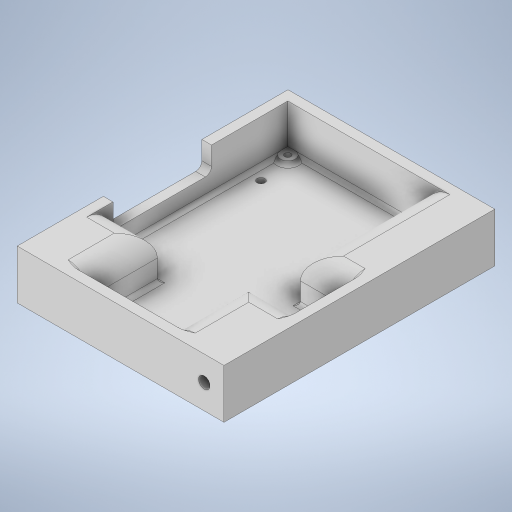
# Autodesk Inventor part: top
Saved by Autodesk Inventor 2024 (Build 280153000, 153)
## iProperties
Created: 2023-11-27
Part Number: top
Material: Generic
Document SubType Name: Modeling
Designer: CJ110
Density: 1 g/cm^3
Appearance: Default
Author: CJ110
Autodesk Inventor part; units mm, degrees
ref_plane "YZ Plane" through (0, 0, 0) normal (1, 0, 0) x (0, 1, 0)
ref_plane "XZ Plane" through (0, 0, 0) normal (0, 1, 0) x (-1, 0, 0)
ref_plane "XY Plane" through (0, 0, 0) normal (0, 0, 1) x (1, 0, 0)
sketch "Sketch1" plane through (0, 0, 0) normal (0, 1, 0) x (-1, 0, 0)
  line L0 (-42.5196, -32.4485) -> (42.5196, -32.4485) construction
  line L1 (42.5196, -32.4485) -> (42.5196, 32.4485) construction
  line L2 (42.5196, 32.4485) -> (-42.5196, 32.4485) construction
  line L3 (-42.5196, 32.4485) -> (-42.5196, -32.4485) construction
  line L4 (-42.5196, -32.4485) -> (42.5196, 32.4485) construction
  line L5 (42.5196, -32.4485) -> (-42.5196, 32.4485) construction
  circle A0 centre (42.5196, 32.4485) radius 3.81
  circle A1 centre (42.5196, 32.4485) radius 1.5875
  circle A2 centre (-42.5196, 32.4485) radius 3.81
  circle A3 centre (-42.5196, 32.4485) radius 1.5875
  circle A4 centre (-42.5196, -32.4485) radius 3.81
  circle A5 centre (-42.5196, -32.4485) radius 1.5875
  circle A6 centre (42.5196, -32.4485) radius 3.81
  circle A7 centre (42.5196, -32.4485) radius 3.81
  circle A8 centre (42.5196, -32.4485) radius 1.5875
  line L6 (45.085, -35.052) -> (-45.085, -35.052) construction
  line L7 (-45.085, -35.052) -> (-45.085, 35.052) construction
  line L8 (-45.085, 35.052) -> (45.085, 35.052) construction
  line L9 (45.085, 35.052) -> (45.085, -35.052) construction
  line L10 (45.085, -35.052) -> (-45.085, 35.052) construction
  line L11 (-45.085, -35.052) -> (45.085, 35.052) construction
  line L12 (-83.185, 60.452) -> (46.3296, 60.452)
  line L13 (46.3296, 60.452) -> (46.3296, -36.2585)
  line L14 (46.3296, -36.2585) -> (-83.185, -36.2585)
  line L15 (-83.185, -36.2585) -> (-83.185, 60.452)
  line L16 (-88.2777, 65.4368) -> (51.4223, 65.4368)
  line L17 (51.4223, 65.4368) -> (51.4223, -41.2433)
  line L18 (51.4223, -41.2433) -> (-88.2777, -41.2433)
  line L19 (-88.2777, -41.2433) -> (-88.2777, 65.4368)
  line L20 (-19.685, 60.452) -> (-19.685, 36.2585)
  line L21 (-46.3296, -10.8585) -> (-83.185, -10.8585)
  line L22 (-42.5196, 36.2585) -> (-42.5196, 60.452)
  line L23 (-46.3296, -10.8585) -> (-46.3296, -36.2585)
  line L24 (-19.685, 36.2585) -> (46.3296, 36.2585)
  line L25 (-42.5196, 32.4485) -> (-46.3296, 32.4485) construction
  line L26 (-42.5196, 32.4485) -> (-42.5196, 36.2585) construction
  line L27 (-46.3296, 32.4485) -> (-83.185, 32.4485)
  line L28 (46.3296, 60.452) -> (51.4223, 60.452) construction
  line L29 (46.3296, 60.452) -> (46.3296, 65.4368) construction
  line L30 (-83.185, -36.2585) -> (-83.185, -41.2433) construction
  line L31 (-83.185, -36.2585) -> (-88.2777, -36.2585) construction
  point P0 (0, 0)
  point P1 (-39.7379, 35.052)
  point P2 (-45.085, 29.6316)
  point P3 (46.3296, 32.4485)
  point P4 (39.7379, 35.052)
  point P5 (-45.085, -29.6316)
  point P6 (-42.5196, -36.2585)
  point P7 (-83.185, 36.2585)
  point P8 (-45.085, 35.2654)
  point P9 (-39.7379, -35.052)
  point P10 (39.7379, -35.052)
  point P11 (45.085, -29.6316)
  point P12 (45.085, 29.6316)
  point P13 (42.5196, -36.2585)
  point P14 (46.3296, -32.4485)
  point P15 (39.7379, 35.052)
  point P16 (-45.085, -29.6316)
  point P17 (-46.3296, -32.4485)
  point P18 (42.5196, 36.2585)
  dimension "d5" = 7.62
  dimension "d7" = 7.62
  dimension "d4" = 7.62
  dimension "d6" = 7.62
  dimension "d8" = 3.175
  dimension "d9" = 3.175
  dimension "d10" = 3.175
  dimension "d11" = 3.175
  dimension "d18" = 70.104
  dimension "d19" = 90.17
  dimension "d23" = 85.0392
  dimension "d24" = 64.897
  dimension "d25" = 38.1
  dimension "d26" = 25.4
  dimension "d31" = 25.4
  dimension "d32" = 25.4
  dimension "d41" = 139.7
  dimension "d43" = 106.68
  constraints: 64 end point, 14 point on line, 13 perpendicular, 10 parallel, 9 coincident, 7 centre point, 6 horizontal, 4 midpoint, 2 point on circle, 2 tangent, 1 collinear, 1 concentric, 1 vertical, 6 other
  measures "d4" diameter of A2
  measures "d6" diameter of A6
  measures "d8" diameter of A3
  measures "d9" diameter of A1
  measures "d10" diameter of A8
  measures "d11" diameter of A5
  measures "d18" distance of L6.end L7.end
  measures "d19" distance of L6.start L6.end
  measures "d23" distance of L1.end L2.end
  measures "d24" distance of L2.end L0.start
  measures "d25" distance between parallel lines of L7 L15
  measures "d26" distance between parallel lines of L8 L12
  measures "d31" distance between parallel lines of L7 L20
  measures "d32" distance between parallel lines of L14 L21
  measures "d41" distance between parallel lines of L17 L19
  measures "d43" distance between parallel lines of L16 L18
extrude "Extrusion5" add sketch "Sketch1" against normal blind 3.175 contours L13 A6 L14 A4 L23 L21 L15 L27 A2 L22 L12 L20 L24 A0 | A0 L24 L13 | L24 L20 L12 L13 | L13 L14 A6 | L14 L23 A4 | L22 A2 L27 L15 L12 | L23 L14 L15 L21 | L16 L17 L18 L19
extrude "Extrusion2" add sketch "Sketch1" against normal blind 5.08 contours A0 | A0 L24 L13 | A6 | L13 L14 A6 | L14 L23 A4 | A4 | A2
extrude "Extrusion4" add sketch "Sketch1" against normal blind 25.4 contours L24 L20 L12 L13 | L22 A2 L27 L15 L12 | L23 L14 L15 L21 | L16 L17 L18 L19
fillet "Fillet1" radius 11.1125 1 edges at (83.185, -3.175, 10.795)
fillet "Fillet2" radius 11.1125 1 edges at (31.1023, -3.175, 60.452)
fillet "Fillet3" radius 11.1125 6 edges at (42.5196, -25.4, 48.3553) (64.7573, -25.4, -10.8585) (46.3296, -25.4, -23.5585) (-13.3223, -25.4, 36.2585) (19.685, -25.4, 48.3552) (64.7573, -25.4, 32.4485)
fillet "Fillet4" radius 1.905 19 edges at (-46.3296, -3.175, 0) (-39.8255, -3.175, -29.7544) (39.8255, -3.175, -29.7544) (46.3296, -3.175, -21.6535) (79.9302, -6.4298, -10.8585) (83.185, -22.1452, -14.1133) (59.2011, -3.175, -10.8585) (-11.4173, -3.175, 36.2585) (19.685, -6.4298, 57.1972) (16.4302, -22.1452, 60.452) (19.685, -3.175, 42.799) (39.8255, -3.175, 29.7544) (42.5196, -6.4298, 57.1972) (45.7744, -22.1452, 60.452) (42.5196, -3.175, 42.799) (79.9302, -6.4298, 32.4485) (59.2011, -3.175, 32.4485) (0, -3.175, -36.2585) (-39.8255, -3.175, 29.7544)
sketch "Sketch4" plane through (0, 0, 0) normal (0, 1, 0) x (1, 0, 0)
  line L0 (88.2777, -65.4368) -> (-51.4223, -65.4368) construction
  line L1 (-51.4223, -65.4368) -> (-51.4223, 41.2433) construction
  line L2 (-51.4223, 41.2433) -> (88.2777, 41.2433) construction
  line L3 (88.2777, 41.2433) -> (88.2777, -65.4368) construction
  line L4 (50.5528, -6.0666) -> (50.5528, -17.9953)
  line L5 (50.5528, -17.9953) -> (48.6146, -18.1269)
  spline S0 degree 2 poles (48.6146, -18.1269) (47.1668, -18.1269) (46.3173, -17.2296) knots 0 0 0 1 1 1
  spline S1 degree 2 poles (46.3173, -17.2296) (45.4798, -16.3203) (45.4798, -14.9324) knots 0 0 0 1 1 1
  spline S2 degree 2 poles (45.4798, -14.9324) (45.4798, -13.1855) (46.9993, -12.4198) knots 0 0 0 1 1 1
  spline S3 degree 2 poles (46.9993, -12.4198) (44.5585, -11.8694) (44.5585, -9.2492) knots 0 0 0 1 1 1
  spline S4 degree 2 poles (44.5585, -9.2492) (44.5585, -7.9211) (45.3602, -6.928) knots 0 0 0 1 1 1
  spline S5 degree 2 poles (45.3602, -6.928) (46.1738, -5.9349) (47.9924, -5.9349) knots 0 0 0 1 1 1
  spline S6 degree 2 poles (47.9924, -5.9349) (48.6505, -5.9349) (49.4401, -6.0067) knots 0 0 0 1 1 1
  spline S7 degree 2 poles (49.4401, -6.0067) (50.1341, -6.0666) (50.5528, -6.0666) knots 0 0 0 1 1 1
  line L6 (48.483, -11.8216) -> (49.6196, -11.8216)
  line L7 (49.6196, -11.8216) -> (49.6196, -9.7876)
  spline S8 degree 2 poles (49.6196, -9.7876) (49.6196, -7.6579) (49.153, -7.0836) knots 0 0 0 1 1 1
  spline S9 degree 2 poles (49.153, -7.0836) (48.7581, -6.7844) (47.9685, -6.7844) knots 0 0 0 1 1 1
  spline S10 degree 2 poles (47.9685, -6.7844) (46.6404, -6.7844) (46.0661, -7.5502) knots 0 0 0 1 1 1
  spline S11 degree 2 poles (46.0661, -7.5502) (45.5277, -8.3159) (45.5277, -9.3449) knots 0 0 0 1 1 1
  spline S12 degree 2 poles (45.5277, -9.3449) (45.5277, -10.1704) (45.8747, -10.7567) knots 0 0 0 1 1 1
  spline S13 degree 2 poles (45.8747, -10.7567) (46.2456, -11.3549) (46.784, -11.5942) knots 0 0 0 1 1 1
  spline S14 degree 2 poles (46.784, -11.5942) (47.3583, -11.8216) (48.483, -11.8216) knots 0 0 0 1 1 1
  line L8 (51.3784, -17.9953) -> (51.3784, -6.0666)
  spline S15 degree 2 poles (51.3784, -6.0666) (52.3715, -6.0307) (53.7594, -5.9349) knots 0 0 0 1 1 1
  line L9 (53.7594, -5.9349) -> (53.7594, -6.1383)
  spline S16 degree 2 poles (53.7594, -6.1383) (52.3116, -6.5332) (52.3116, -9.2013) knots 0 0 0 1 1 1
  line L10 (52.3116, -9.2013) -> (52.3116, -15.0999)
  spline S17 degree 2 poles (52.3116, -15.0999) (52.3116, -17.445) (53.7594, -17.9235) knots 0 0 0 1 1 1
  line L11 (53.7594, -17.9235) -> (53.7594, -18.1269)
  spline S18 degree 2 poles (53.7594, -18.1269) (52.5868, -18.0193) (51.3784, -17.9953) knots 0 0 0 1 1 1
  line L12 (49.6196, -14.8965) -> (49.6196, -12.6232)
  line L13 (49.6196, -12.6232) -> (48.7462, -12.6232)
  spline S19 degree 2 poles (48.7462, -12.6232) (47.6574, -12.6232) (47.0711, -13.2095) knots 0 0 0 1 1 1
  spline S20 degree 2 poles (47.0711, -13.2095) (46.4729, -13.7957) (46.4729, -14.9084) knots 0 0 0 1 1 1
  spline S21 degree 2 poles (46.4729, -14.9084) (46.4729, -16.0571) (47.119, -16.6553) knots 0 0 0 1 1 1
  spline S22 degree 2 poles (47.119, -16.6553) (47.7531, -17.2416) (48.6385, -17.2416) knots 0 0 0 1 1 1
  spline S23 degree 2 poles (48.6385, -17.2416) (49.1171, -17.2416) (49.4162, -17.0023) knots 0 0 0 1 1 1
  spline S24 degree 2 poles (49.4162, -17.0023) (49.6196, -16.3921) (49.6196, -14.8965) knots 0 0 0 1 1 1
  spline S25 degree 2 poles (44.7619, -6.3896) (43.721, -7.4784) (43.721, -9.1893) knots 0 0 0 1 1 1
  spline S26 degree 2 poles (43.721, -9.1893) (43.721, -11.0199) (44.8098, -12.1446) knots 0 0 0 1 1 1
  spline S27 degree 2 poles (44.8098, -12.1446) (42.6562, -11.3669) (42.6562, -9.2851) knots 0 0 0 1 1 1
  spline S28 degree 2 poles (42.6562, -9.2851) (42.6562, -8.2561) (43.2544, -7.4545) knots 0 0 0 1 1 1
  spline S29 degree 2 poles (43.2544, -7.4545) (43.8526, -6.6528) (44.7619, -6.3896) knots 0 0 0 1 1 1
  spline S30 degree 2 poles (45.3243, -12.7787) (44.6303, -13.6881) (44.6303, -14.9324) knots 0 0 0 1 1 1
  spline S31 degree 2 poles (44.6303, -14.9324) (44.6303, -15.9135) (45.0132, -16.7031) knots 0 0 0 1 1 1
  spline S32 degree 2 poles (45.0132, -16.7031) (45.42, -17.5048) (45.9345, -17.78) knots 0 0 0 1 1 1
  spline S33 degree 2 poles (45.9345, -17.78) (44.8098, -17.5407) (44.2116, -16.8108) knots 0 0 0 1 1 1
  spline S34 degree 2 poles (44.2116, -16.8108) (43.6133, -16.081) (43.6133, -15.1836) knots 0 0 0 1 1 1
  spline S35 degree 2 poles (43.6133, -15.1836) (43.6133, -14.394) (44.1158, -13.6881) knots 0 0 0 1 1 1
  spline S36 degree 2 poles (44.1158, -13.6881) (44.6064, -13.0061) (45.3243, -12.7787) knots 0 0 0 1 1 1
  spline S37 degree 2 poles (29.5189, -12.0968) (29.5189, -10.0029) (30.1531, -8.5672) knots 0 0 0 1 1 1
  spline S38 degree 2 poles (30.1531, -8.5672) (30.7752, -7.1434) (31.9119, -6.4614) knots 0 0 0 1 1 1
  spline S39 degree 2 poles (31.9119, -6.4614) (33.0126, -5.7674) (34.4963, -5.7674) knots 0 0 0 1 1 1
  spline S40 degree 2 poles (34.4963, -5.7674) (36.8533, -5.7674) (38.1455, -7.4545) knots 0 0 0 1 1 1
  spline S41 degree 2 poles (38.1455, -7.4545) (39.4377, -9.1415) (39.4377, -12.0968) knots 0 0 0 1 1 1
  spline S42 degree 2 poles (39.4377, -12.0968) (39.4377, -15.1717) (38.1215, -16.8108) knots 0 0 0 1 1 1
  spline S43 degree 2 poles (38.1215, -16.8108) (36.8054, -18.4261) (34.5202, -18.4261) knots 0 0 0 1 1 1
  spline S44 degree 2 poles (34.5202, -18.4261) (32.211, -18.4261) (30.859, -16.8108) knots 0 0 0 1 1 1
  spline S45 degree 2 poles (30.859, -16.8108) (29.5189, -15.2076) (29.5189, -12.0968) knots 0 0 0 1 1 1
  spline S46 degree 2 poles (30.5838, -12.0848) (30.5838, -17.5048) (34.5202, -17.5048) knots 0 0 0 1 1 1
  spline S47 degree 2 poles (34.5202, -17.5048) (38.3848, -17.5048) (38.3848, -11.9412) knots 0 0 0 1 1 1
  spline S48 degree 2 poles (38.3848, -11.9412) (38.3848, -6.7126) (34.4843, -6.7126) knots 0 0 0 1 1 1
  spline S49 degree 2 poles (34.4843, -6.7126) (30.5838, -6.7126) (30.5838, -12.0848) knots 0 0 0 1 1 1
  spline S50 degree 2 poles (39.0548, -16.9424) (40.2991, -15.0161) (40.2991, -12.013) knots 0 0 0 1 1 1
  spline S51 degree 2 poles (40.2991, -12.013) (40.2991, -9.297) (39.1146, -7.2989) knots 0 0 0 1 1 1
  spline S52 degree 2 poles (39.1146, -7.2989) (41.3999, -8.8065) (41.3999, -12.1207) knots 0 0 0 1 1 1
  spline S53 degree 2 poles (41.3999, -12.1207) (41.3999, -15.5306) (39.0548, -16.9424) knots 0 0 0 1 1 1
  spline S54 degree 2 poles (29.9257, -7.2391) (28.6934, -8.9141) (28.6934, -12.2882) knots 0 0 0 1 1 1
  spline S55 degree 2 poles (28.6934, -12.2882) (28.6934, -15.2674) (29.9138, -16.9305) knots 0 0 0 1 1 1
  spline S56 degree 2 poles (29.9138, -16.9305) (27.5926, -15.5306) (27.5926, -12.1566) knots 0 0 0 1 1 1
  spline S57 degree 2 poles (27.5926, -12.1566) (27.5926, -8.8304) (29.9257, -7.2391) knots 0 0 0 1 1 1
  line L14 (19.1336, -6.0666) -> (19.4208, -6.0666)
  line L15 (19.4208, -6.0666) -> (19.4208, -17.9953)
  line L16 (19.4208, -17.9953) -> (15.3528, -17.9953)
  spline S58 degree 2 poles (15.3528, -17.9953) (14.2281, -17.9953) (13.1513, -18.1269) knots 0 0 0 1 1 1
  spline S59 degree 2 poles (13.1513, -18.1269) (13.1513, -17.9116) (13.1752, -17.3492) knots 0 0 0 1 1 1
  spline S60 degree 2 poles (13.1752, -17.3492) (13.2111, -16.8348) (13.2111, -16.0451) knots 0 0 0 1 1 1
  spline S61 degree 2 poles (13.2111, -16.0451) (13.2111, -15.5545) (13.2709, -15.0401) knots 0 0 0 1 1 1
  line L17 (13.2709, -15.0401) -> (13.5461, -15.0401)
  spline S62 degree 2 poles (13.5461, -15.0401) (13.57, -15.9733) (14.0008, -16.5835) knots 0 0 0 1 1 1
  spline S63 degree 2 poles (14.0008, -16.5835) (14.4554, -17.2057) (15.9151, -17.2057) knots 0 0 0 1 1 1
  line L18 (15.9151, -17.2057) -> (18.4875, -17.2057)
  line L19 (18.4875, -17.2057) -> (18.4875, -9.1056)
  spline S64 degree 2 poles (18.4875, -9.1056) (18.4875, -7.7057) (18.0927, -7.0118) knots 0 0 0 1 1 1
  spline S65 degree 2 poles (18.0927, -7.0118) (17.6979, -6.3058) (16.8723, -6.1383) knots 0 0 0 1 1 1
  line L20 (16.8723, -6.1383) -> (16.8723, -5.9349)
  spline S66 degree 2 poles (16.8723, -5.9349) (18.8704, -6.0666) (19.1336, -6.0666) knots 0 0 0 1 1 1
  line L21 (23.9913, -17.9953) -> (20.2583, -17.9953)
  line L22 (20.2583, -17.9953) -> (20.2583, -6.0666)
  line L23 (20.2583, -6.0666) -> (20.6053, -6.0666)
  spline S67 degree 2 poles (20.6053, -6.0666) (21.3351, -6.0666) (22.7948, -5.9349) knots 0 0 0 1 1 1
  line L24 (22.7948, -5.9349) -> (22.7948, -6.1383)
  spline S68 degree 2 poles (22.7948, -6.1383) (21.8616, -6.3776) (21.5026, -7.0955) knots 0 0 0 1 1 1
  spline S69 degree 2 poles (21.5026, -7.0955) (21.1676, -7.8134) (21.1676, -9.4765) knots 0 0 0 1 1 1
  line L25 (21.1676, -9.4765) -> (21.1676, -17.2057)
  line L26 (21.1676, -17.2057) -> (24.0511, -17.2057)
  spline S70 degree 2 poles (24.0511, -17.2057) (25.1518, -17.2057) (25.6065, -16.751) knots 0 0 0 1 1 1
  spline S71 degree 2 poles (25.6065, -16.751) (26.0612, -16.2964) (26.3603, -15.0401) knots 0 0 0 1 1 1
  line L27 (26.3603, -15.0401) -> (26.6235, -15.0401)
  spline S72 degree 2 poles (26.6235, -15.0401) (26.6355, -15.1956) (26.6355, -15.3631) knots 0 0 0 1 1 1
  spline S73 degree 2 poles (26.6355, -15.3631) (26.6355, -15.5904) (26.5876, -15.9374) knots 0 0 0 1 1 1
  spline S74 degree 2 poles (26.5876, -15.9374) (26.456, -17.1458) (26.456, -18.1269) knots 0 0 0 1 1 1
  spline S75 degree 2 poles (26.456, -18.1269) (25.8578, -18.0552) (24.9604, -18.0312) knots 0 0 0 1 1 1
  line L28 (24.9604, -18.0312) -> (23.9913, -17.9953)
  line L29 (4.8837, -6.0666) -> (5.1708, -6.0666)
  line L30 (5.1708, -6.0666) -> (5.1708, -17.9953)
  line L31 (5.1708, -17.9953) -> (1.1029, -17.9953)
  spline S76 degree 2 poles (1.1029, -17.9953) (-0.0218, -17.9953) (-1.0986, -18.1269) knots 0 0 0 1 1 1
  spline S77 degree 2 poles (-1.0986, -18.1269) (-1.0986, -17.9116) (-1.0747, -17.3492) knots 0 0 0 1 1 1
  spline S78 degree 2 poles (-1.0747, -17.3492) (-1.0388, -16.8348) (-1.0388, -16.0451) knots 0 0 0 1 1 1
  spline S79 degree 2 poles (-1.0388, -16.0451) (-1.0388, -15.5545) (-0.979, -15.0401) knots 0 0 0 1 1 1
  line L32 (-0.979, -15.0401) -> (-0.7038, -15.0401)
  spline S80 degree 2 poles (-0.7038, -15.0401) (-0.6799, -15.9733) (-0.2492, -16.5835) knots 0 0 0 1 1 1
  spline S81 degree 2 poles (-0.2492, -16.5835) (0.2055, -17.2057) (1.6652, -17.2057) knots 0 0 0 1 1 1
  line L33 (1.6652, -17.2057) -> (4.2376, -17.2057)
  line L34 (4.2376, -17.2057) -> (4.2376, -9.1056)
  spline S82 degree 2 poles (4.2376, -9.1056) (4.2376, -7.7057) (3.8428, -7.0118) knots 0 0 0 1 1 1
  spline S83 degree 2 poles (3.8428, -7.0118) (3.4479, -6.3058) (2.6224, -6.1383) knots 0 0 0 1 1 1
  line L35 (2.6224, -6.1383) -> (2.6224, -5.9349)
  spline S84 degree 2 poles (2.6224, -5.9349) (4.6205, -6.0666) (4.8837, -6.0666) knots 0 0 0 1 1 1
  line L36 (9.7413, -17.9953) -> (6.0084, -17.9953)
  line L37 (6.0084, -17.9953) -> (6.0084, -6.0666)
  line L38 (6.0084, -6.0666) -> (6.3553, -6.0666)
  spline S85 degree 2 poles (6.3553, -6.0666) (7.0852, -6.0666) (8.5449, -5.9349) knots 0 0 0 1 1 1
  line L39 (8.5449, -5.9349) -> (8.5449, -6.1383)
  spline S86 degree 2 poles (8.5449, -6.1383) (7.6116, -6.3776) (7.2527, -7.0955) knots 0 0 0 1 1 1
  spline S87 degree 2 poles (7.2527, -7.0955) (6.9177, -7.8134) (6.9177, -9.4765) knots 0 0 0 1 1 1
  line L40 (6.9177, -9.4765) -> (6.9177, -17.2057)
  line L41 (6.9177, -17.2057) -> (9.8012, -17.2057)
  spline S88 degree 2 poles (9.8012, -17.2057) (10.9019, -17.2057) (11.3566, -16.751) knots 0 0 0 1 1 1
  spline S89 degree 2 poles (11.3566, -16.751) (11.8112, -16.2964) (12.1104, -15.0401) knots 0 0 0 1 1 1
  line L42 (12.1104, -15.0401) -> (12.3736, -15.0401)
  spline S90 degree 2 poles (12.3736, -15.0401) (12.3855, -15.1956) (12.3855, -15.3631) knots 0 0 0 1 1 1
  spline S91 degree 2 poles (12.3855, -15.3631) (12.3855, -15.5904) (12.3377, -15.9374) knots 0 0 0 1 1 1
  spline S92 degree 2 poles (12.3377, -15.9374) (12.2061, -17.1458) (12.2061, -18.1269) knots 0 0 0 1 1 1
  spline S93 degree 2 poles (12.2061, -18.1269) (11.6078, -18.0552) (10.7105, -18.0312) knots 0 0 0 1 1 1
  line L43 (10.7105, -18.0312) -> (9.7413, -17.9953)
  line L44 (-10.6943, -6.0666) -> (-10.6943, -12.0968)
  line L45 (-10.6943, -12.0968) -> (-5.035, -17.9953)
  line L46 (-5.035, -17.9953) -> (-5.3581, -17.9953)
  spline S94 degree 2 poles (-5.3581, -17.9953) (-6.6981, -17.9953) (-8.1458, -18.1269) knots 0 0 0 1 1 1
  line L47 (-8.1458, -18.1269) -> (-8.1458, -17.9235)
  spline S95 degree 2 poles (-8.1458, -17.9235) (-7.4758, -17.7321) (-7.4758, -17.2894) knots 0 0 0 1 1 1
  spline S96 degree 2 poles (-7.4758, -17.2894) (-7.4758, -16.7031) (-8.8278, -15.2913) knots 0 0 0 1 1 1
  line L48 (-8.8278, -15.2913) -> (-11.2208, -12.7907)
  line L49 (-11.2208, -12.7907) -> (-13.4582, -15.399)
  spline S97 degree 2 poles (-13.4582, -15.399) (-14.2, -16.2724) (-14.2, -16.9664) knots 0 0 0 1 1 1
  spline S98 degree 2 poles (-14.2, -16.9664) (-14.2, -17.7441) (-13.4223, -17.9235) knots 0 0 0 1 1 1
  line L50 (-13.4223, -17.9235) -> (-13.4223, -18.1269)
  spline S99 degree 2 poles (-13.4223, -18.1269) (-13.6974, -18.1269) (-14.7982, -18.0432) knots 0 0 0 1 1 1
  spline S100 degree 2 poles (-14.7982, -18.0432) (-15.2648, -17.9953) (-15.6238, -17.9953) knots 0 0 0 1 1 1
  spline S101 degree 2 poles (-15.6238, -17.9953) (-15.8152, -17.9953) (-17.6099, -18.1269) knots 0 0 0 1 1 1
  line L51 (-17.6099, -18.1269) -> (-17.6099, -17.9235)
  spline S102 degree 2 poles (-17.6099, -17.9235) (-16.7604, -17.6723) (-16.234, -17.2296) knots 0 0 0 1 1 1
  spline S103 degree 2 poles (-16.234, -17.2296) (-15.7195, -16.7869) (-15.0614, -15.9972) knots 0 0 0 1 1 1
  spline S104 degree 2 poles (-15.0614, -15.9972) (-15.0255, -15.9374) (-14.9059, -15.7938) knots 0 0 0 1 1 1
  line L52 (-14.9059, -15.7938) -> (-11.6156, -11.9532)
  line L53 (-11.6156, -11.9532) -> (-11.6156, -9.0817)
  spline S105 degree 2 poles (-11.6156, -9.0817) (-11.6156, -6.4614) (-13.2428, -6.1383) knots 0 0 0 1 1 1
  line L54 (-13.2428, -6.1383) -> (-13.2428, -5.9349)
  spline S106 degree 2 poles (-13.2428, -5.9349) (-11.1729, -6.0666) (-11.1011, -6.0666) knots 0 0 0 1 1 1
  line L55 (-11.1011, -6.0666) -> (-10.6943, -6.0666)
  line L56 (-3.9582, -17.9953) -> (-9.8209, -11.7737)
  line L57 (-9.8209, -11.7737) -> (-9.8209, -6.0666)
  line L58 (-9.8209, -6.0666) -> (-9.5577, -6.0666)
  spline S107 degree 2 poles (-9.5577, -6.0666) (-8.5646, -6.0666) (-7.2844, -5.9349) knots 0 0 0 1 1 1
  line L59 (-7.2844, -5.9349) -> (-7.2844, -6.1383)
  spline S108 degree 2 poles (-7.2844, -6.1383) (-8.0262, -6.3058) (-8.4569, -6.8802) knots 0 0 0 1 1 1
  spline S109 degree 2 poles (-8.4569, -6.8802) (-8.8757, -7.4425) (-8.8757, -9.0338) knots 0 0 0 1 1 1
  line L60 (-8.8757, -9.0338) -> (-8.8757, -11.5105)
  line L61 (-8.8757, -11.5105) -> (-5.2743, -15.3152)
  spline S110 degree 2 poles (-5.2743, -15.3152) (-3.2164, -17.4689) (-1.5533, -17.9235) knots 0 0 0 1 1 1
  line L62 (-1.5533, -17.9235) -> (-1.5533, -18.1269)
  spline S111 degree 2 poles (-1.5533, -18.1269) (-2.4985, -17.9953) (-3.5873, -17.9953) knots 0 0 0 1 1 1
  line L63 (-3.5873, -17.9953) -> (-3.9582, -17.9953)
  point P0 (0, 0)
  constraints: 2 coincident, 2 other
emboss "Emboss1" sketch "Sketch4" operation cut depth 0.4 direction (0, -1, 0)
sketch "Sketch5" plane through (0, 0, 0) normal (0, 1, 0) x (1, 0, 0)
  line L0 (40.6146, -49.3395) -> (40.6146, -37.8367) projected
  line L1 (21.59, -49.3395) -> (40.6146, -49.3395) projected
  line L2 (21.59, -34.3535) -> (21.59, -49.3395) projected
  line L3 (-37.1314, -34.3535) -> (21.59, -34.3535) projected
  arc A0 (-37.1314, -34.3535) -> (-44.4246, -27.0603) centre (-42.5196, -32.4485) ccw projected
  line L4 (-44.4246, 27.0603) -> (-44.4246, -27.0603) projected
  arc A1 (-44.4246, 27.0603) -> (-37.1314, 34.3535) centre (-42.5196, 32.4485) ccw projected
  line L5 (37.1314, 34.3535) -> (-37.1314, 34.3535) projected
  arc A2 (37.1314, 34.3535) -> (44.4246, 27.0603) centre (42.5196, 32.4485) ccw projected
  line L6 (44.4246, 8.9535) -> (44.4246, 27.0603) projected
  line L7 (72.0725, 8.9535) -> (44.4246, 8.9535) projected
  line L8 (72.0725, -30.5435) -> (72.0725, 8.9535) projected
  line L9 (47.9078, -30.5435) -> (72.0725, -30.5435) projected
  arc A3 (47.9078, -30.5435) -> (40.6146, -37.8367) centre (42.5196, -32.4485) ccw projected
  circle A4 centre (-26.0223, 29.8133) radius 2.032
  circle A5 centre (62.8777, 29.8133) radius 3
  line L10 (-51.4223, 41.2433) -> (-51.4223, -65.4368) projected
  line L11 (88.2777, 41.2433) -> (-51.4223, 41.2433) projected
  line L12 (88.2777, -65.4368) -> (88.2777, 41.2433) projected
  point P0 (0, 0)
  dimension "d60" = 4.064
  dimension "d61" = 6
  dimension "d62" = 25.4
  dimension "d63" = 11.43
  dimension "d64" = 25.4
  dimension "d65" = 11.43
  constraints: 2 centre point
  measures "d60" diameter of A4
  measures "d61" diameter of A5
  measures "d62" distance from line of L10 A4.centre
  measures "d63" distance from line of L11 A4.centre
  measures "d64" distance from line of L12 A5.centre
  measures "d65" distance from line of L11 A5.centre
extrude "Extrusion8" cut sketch "Sketch5" against normal blind 11 contours A4 | A5
sketch "Sketch6" plane through (88.2777, 0, -41.2433) normal (0, 0, -1) x (-1, 0, 0)
  line L0 (0, 0) -> (139.7, 0) projected
  line L1 (0, 0) -> (0, -25.4) projected
  line L2 (139.7, -25.4) -> (0, -25.4) projected
  line L3 (139.7, 0) -> (139.7, -25.4) projected
  line L4 (44.45, -25.4) -> (95.25, -25.4)
  line L5 (95.25, -25.4) -> (95.25, -12.7)
  line L6 (95.25, -12.7) -> (44.45, -12.7)
  line L7 (44.45, -12.7) -> (44.45, -25.4)
  line L8 (69.85, 0) -> (69.85, -25.4) construction
  point P0 (88.2777, 0)
  dimension "d68" = 50.8
  dimension "d69" = 12.7
  constraints: 10 end point, 2 midpoint, 2 parallel, 1 horizontal, 1 perpendicular, 1 point on line, 1 vertical
  measures "d68" distance of L5.end L6.end
  measures "d69" distance between parallel lines of L2 L6
extrude "Extrusion9" cut sketch "Sketch6" against normal up to surface (4.9848 mm away) contours L7 L6 L5 L2
fillet "Fillet5" radius 3.175 2 edges at (43.8277, -12.7, -38.7509) (-6.9723, -12.7, -38.7509)
sketch "Sketch7" plane through (88.2777, 0, 65.4368) normal (1, 0, 0) x (0, 0, -1)
  line L0 (0, 0) -> (106.68, 0) projected
  line L1 (0, 0) -> (0, -25.4) projected
  line L2 (106.68, -25.4) -> (0, -25.4) projected
  line L3 (106.68, 0) -> (106.68, -25.4) projected
  circle A0 centre (10.16, -12.7) radius 3
  line L4 (0, -12.7) -> (106.68, -12.7) construction
  point P0 (65.4368, 0)
  dimension "d73" = 6
  dimension "d74" = 10.16
  constraints: 2 end point, 2 midpoint, 1 centre point, 1 point on line
  measures "d73" diameter of A0
  measures "d74" distance from line of L1 A0.centre
extrude "Extrusion10" cut sketch "Sketch7" against normal blind 11 contours A0
ref_plane "Work Plane1" through (-51.4223, 0, 12.0967) normal (0, 0, 1) x (1, 0, 0)
ref_plane "Work Plane2" through (18.4277, 0, -41.2433) normal (-1, 0, 0) x (0, 0, 1)
mirror "Mirror4" about plane through (18.4277, 0, -41.2433) normal (-1, 0, 0) of "Extrusion10"
sketch "Sketch2" plane through (0, -25.4, 0) normal (0, -1, 0) x (1, 0, 0)
  circle A0 centre (-53.9623, -34.8933) radius 1.27
  arc A1 (-53.9623, -31.0833) -> (-53.9623, -38.7033) centre (-53.9623, -34.8933) ccw
  line L0 (83.185, 36.7811) -> (83.185, -15.1911) projected
  line L1 (57.4421, -21.971) -> (81.28, -21.971) projected
  line L2 (57.4421, -36.2585) -> (57.4421, -21.971) projected
  line L3 (-6.9723, -36.2585) -> (-46.3296, -36.2585) projected
  line L4 (-46.3296, -36.2585) -> (-46.3296, 47.371) projected
  line L5 (8.5725, 47.371) -> (-46.3296, 47.371) projected
  line L6 (8.5725, 58.547) -> (8.5725, 47.371) projected
  line L7 (15.3524, 60.452) -> (46.8522, 60.452) projected
  line L8 (53.6321, 43.561) -> (53.6321, 58.547) projected
  line L9 (81.28, 43.561) -> (53.6321, 43.561) projected
  line L10 (-51.4223, -41.2433) -> (-6.9723, -41.2433) projected
  line L11 (88.2777, -41.2433) -> (88.2777, 65.4368) projected
  line L12 (88.2777, 65.4368) -> (-51.4223, 65.4368) projected
  line L13 (-51.4223, 65.4368) -> (-51.4223, -41.2433) projected
  line L14 (-51.4223, -31.0833) -> (-53.9623, -31.0833)
  line L15 (-51.4223, -41.2433) -> (-51.4223, 65.4368) projected
  line L16 (-51.4223, -38.7033) -> (-53.9623, -38.7033)
  line L17 (-6.9723, -41.2433) -> (-6.9723, -36.2585) projected
  line L18 (57.4421, -36.2585) -> (43.8277, -36.2585) projected
  line L19 (43.8277, -36.2585) -> (43.8277, -41.2433) projected
  line L20 (43.8277, -41.2433) -> (88.2777, -41.2433) projected
  point P0 (0, 0)
  point P1 (-51.4223, -38.7033)
  dimension "d45" = 2.54
  dimension "d46" = 7.62
  dimension "d51" = 2.54
  dimension "d53" = 2.54
  constraints: 4 end point, 2 centre point, 2 point on circle, 2 point on line, 2 tangent, 1 coincident, 1 horizontal, 1 perpendicular, 4 other
  measures "d45" diameter of A0
  measures "d46" diameter of A1
  measures "d51" distance from line of L13 A0.centre
  measures "d53" distance between parallel lines of L16 L10
sketch "Sketch3" plane through (88.2777, 0, 65.4368) normal (1, 0, 0) x (0, 0, -1)
  circle A0 centre (10.16, -12.7) radius 3
  line L0 (96.52, -25.4) -> (96.52, -22.225) projected
  line L1 (96.52, -22.225) -> (104.14, -22.225) projected
  line L2 (104.14, -22.225) -> (104.14, -25.4) projected
  line L3 (106.68, -25.4) -> (104.14, -25.4) projected
  line L4 (106.68, 0) -> (106.68, -25.4) projected
  line L5 (0, 0) -> (106.68, 0) projected
  line L6 (0, 0) -> (0, -25.4) projected
  line L7 (96.52, -25.4) -> (0, -25.4) projected
  line L8 (106.68, -12.7) -> (0, -12.7) construction
  point P0 (65.4368, 0)
  dimension "d54" = 6
  dimension "d55" = 10.16
  constraints: 2 end point, 2 midpoint, 1 centre point, 1 point on line
  measures "d54" diameter of A0
  measures "d55" distance from line of L6 A0.centre
equation "\"d5\" = d4"
equation "\"d7\" = d4"
equation "\"d6\" = d4"
equation "\"d9\" = d8"
equation "\"d10\" = d8"
equation "\"d11\" = d8"
body "Solid1"
